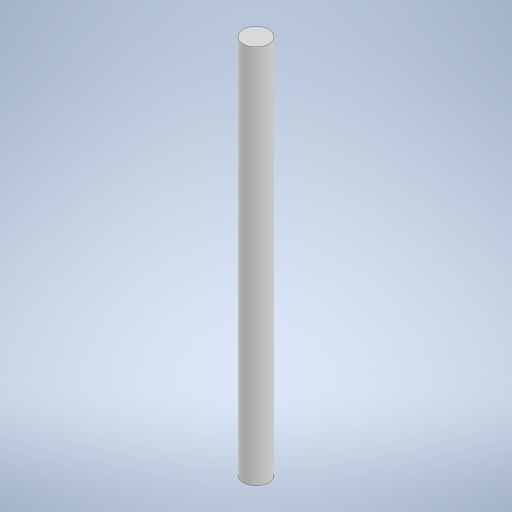
# Autodesk Inventor part: bore template
Saved by Autodesk Inventor 2023 (Build 270158000, 158)
## iProperties
Created: 2023-03-02
Part Number: bore template
Material: Generic
Document SubType Name: Modeling
Designer: dncob
Density: 1 g/cm^3
Appearance: Default
Author: dncob
Autodesk Inventor part; units mm, degrees
ref_plane "YZ Plane" through (0, 0, 0) normal (1, 0, 0) x (0, 1, 0)
ref_plane "XZ Plane" through (0, 0, 0) normal (0, 1, 0) x (-1, 0, 0)
ref_plane "XY Plane" through (0, 0, 0) normal (0, 0, 1) x (1, 0, 0)
sketch "bore revolve" plane through (0, 0, 0) normal (0, 0, 1) x (1, 0, 0)
  line L0 (12.7, 381) -> (0, 381)
  line L1 (12.7, 0) -> (0, 0)
  line L2 (0, 0) -> (0, 381)
  spline S0 degree 4 poles (12.7, 381) (12.7, 369.0938) (12.7, 352.425) (12.7, 330.9937) (12.7, 304.8) (12.7, 285.75) (12.7, 266.7) (12.7, 247.65) (12.7, 228.6) (12.7, 209.55) (12.7, 190.5) (12.7, 171.45) (12.7, 152.4) (12.7, 133.35) (12.7, 114.3) (12.7, 95.25) (12.7, 76.2) (12.7, 50.0062) (12.7, 28.575) (12.7, 11.9063) (12.7, 0) knots 0 0 0 0 0 0.125 0.175 0.225 0.275 0.325 0.375 0.425 0.475 0.525 0.575 0.625 0.675 0.725 0.775 0.825 0.875 1 1 1 1 1
  point P0 (0, 19.05)
  point P1 (0, 38.1)
  point P2 (0, 57.15)
  point P3 (0, 76.2)
  point P4 (0, 95.25)
  point P5 (0, 114.3)
  point P6 (0, 133.35)
  point P7 (0, 152.4)
  point P8 (0, 171.45)
  point P9 (0, 190.5)
  point P10 (0, 209.55)
  point P11 (0, 228.6)
  point P12 (0, 247.65)
  point P13 (0, 266.7)
  point P14 (0, 285.75)
  point P15 (0, 304.8)
  point P16 (0, 323.85)
  point P17 (0, 342.9)
  point P18 (0, 361.95)
  point P19 (0, 381)
  point P20 (12.7, 361.95)
  point P21 (12.7, 342.9)
  point P22 (12.7, 323.85)
  point P23 (12.7, 304.8)
  point P24 (12.7, 285.75)
  point P25 (12.7, 266.7)
  point P26 (12.7, 247.65)
  point P27 (12.7, 228.6)
  point P28 (12.7, 209.55)
  point P29 (12.7, 190.5)
  point P30 (12.7, 171.45)
  point P31 (12.7, 152.4)
  point P32 (12.7, 133.35)
  point P33 (12.7, 114.3)
  point P34 (12.7, 95.25)
  point P35 (12.7, 76.2)
  point P36 (12.7, 57.15)
  point P37 (12.7, 38.1)
  point P38 (12.7, 19.05)
  point P39 (0, 190.5)
  dimension "r0" = 12.7
  dimension "x" = 381
  dimension "d5" = 19.05
  dimension "d11" = 19.05
  dimension "r1" = 12.7
  dimension "r2" = 12.7
  dimension "r3" = 12.7
  dimension "r4" = 12.7
  dimension "r5" = 12.7
  dimension "r6" = 12.7
  dimension "r7" = 12.7
  dimension "r8" = 12.7
  dimension "r9" = 12.7
  dimension "r10" = 12.7
  dimension "r11" = 12.7
  dimension "r12" = 12.7
  dimension "r13" = 12.7
  dimension "r14" = 12.7
  dimension "r15" = 12.7
  dimension "r16" = 12.7
  dimension "r17" = 12.7
  dimension "r18" = 12.7
  dimension "r19" = 12.7
  dimension "r20" = 12.7
  constraints: 19 horizontal alignment, 6 end point, 2 horizontal, 2 vertical, 1 midpoint, 1 point on line, 40 other
  measures "r0" distance from line of L2 L0.start
  measures "x" distance of L1.end L0.end
  measures "d5" distance of point (0, 19.05) point (0, 38.1)
  measures "d11" distance of L1.end point (0, 19.05)
  measures "r1" distance of point (12.7, 361.95) point (0, 361.95)
  measures "r2" distance of point (0, 342.9) point (12.7, 342.9)
  measures "r3" distance of point (0, 323.85) point (12.7, 323.85)
  measures "r4" distance of point (0, 304.8) point (12.7, 304.8)
  measures "r5" distance of point (0, 285.75) point (12.7, 285.75)
  measures "r6" distance of point (0, 266.7) point (12.7, 266.7)
  measures "r7" distance of point (0, 247.65) point (12.7, 247.65)
  measures "r8" distance of point (12.7, 228.6) point (0, 228.6)
  measures "r9" distance of point (0, 209.55) point (12.7, 209.55)
  measures "r10" distance of point (0, 190.5) point (12.7, 190.5)
  measures "r11" distance of point (0, 171.45) point (12.7, 171.45)
  measures "r12" distance of point (0, 152.4) point (12.7, 152.4)
  measures "r13" distance of point (0, 133.35) point (12.7, 133.35)
  measures "r14" distance of point (0, 114.3) point (12.7, 114.3)
  measures "r15" distance of point (0, 95.25) point (12.7, 95.25)
  measures "r16" distance of point (0, 76.2) point (12.7, 76.2)
  measures "r17" distance of point (0, 57.15) point (12.7, 57.15)
  measures "r18" distance of point (12.7, 38.1) point (0, 38.1)
  measures "r19" distance of point (0, 19.05) point (12.7, 19.05)
  measures "r20" distance of L1.end L1.start
revolve "Revolution1" add sketch "bore revolve" angle 360 about axis through (0, 0, 0) along (0, 1, 0)
equation "\"d5\" = 0.05 * x"
equation "\"d11\" = 0.05 * x"
body "Solid1"
